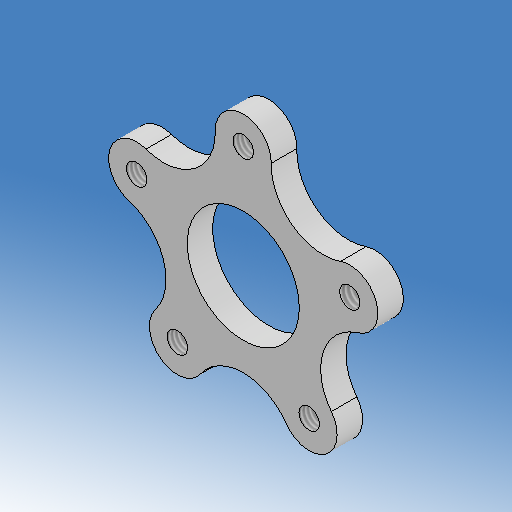
# Autodesk Inventor part: panel_flange
Saved by Autodesk Inventor 2025 (Build 290162000, 162)
## iProperties
Created: 2023-11-12
Part Number: panel_flange
Material: Generic
Document SubType Name: Modeling
Designer: ralph
Density: 1 g/cm^3
Appearance: Default
Author: ralph
Autodesk Inventor part; units mm, degrees
ref_plane "YZ Plane" through (0, 0, 0) normal (1, 0, 0) x (0, 1, 0)
ref_plane "XZ Plane" through (0, 0, 0) normal (0, 1, 0) x (-1, 0, 0)
ref_plane "XY Plane" through (0, 0, 0) normal (0, 0, 1) x (1, 0, 0)
sketch "Sketch1" plane through (0, 0, 0) normal (0, 0, 1) x (1, 0, 0)
  circle A0 centre (0, 0) radius 13.97
  circle A1 centre (0, 0) radius 34.925
  circle A2 centre (0, 0) radius 27.94
  point P0 (0, 27.94)
  point P1 (-26.5725, 8.6339)
  point P2 (-16.4227, -22.6039)
  point P3 (16.4227, -22.6039)
  point P4 (26.5725, 8.6339)
  dimension "d2" = 55.88
  dimension "d0" = 27.94
  dimension "d1" = 69.85
  dimension "d5" = 360
  constraints: 5 coincident, 2 centre point, 1 vertical alignment, 11 other
  measures "d0" diameter of A0
  measures "d1" diameter of A1
extrude "Extrusion1" add sketch "Sketch1" along normal blind 6.35 contours A1 | A2
hole "Hole1" at (0, 27.94, 0) at (-26.5725, 8.6339, 0) at (-16.4227, -22.6039, 0) at (16.4227, -22.6039, 0) at (26.5725, 8.6339, 0) direction (0, 0, 1) diameter 5.1054 end through all
thread "Thread1" size "1/4-20 UNC" class "2B" standard "ANSI Unified Screw Threads" full length
thread "Thread2" size "12-24 UNC" class "2B" standard "ANSI Unified Screw Threads" full length
thread "Thread3" size "12-24 UNC" class "2B" standard "ANSI Unified Screw Threads" full length
thread "Thread4" size "12-24 UNC" class "2B" standard "ANSI Unified Screw Threads" full length
thread "Thread5" size "12-24 UNC" class "2B" standard "ANSI Unified Screw Threads" full length
sketch "Sketch2" plane through (0, 0, 6.35) normal (0, 0, 1) x (1, 0, 0)
  circle A0 centre (0, 27.94) radius 2.5527 projected
  circle A1 centre (-26.5725, 8.6339) radius 2.5527 projected
  circle A2 centre (-16.4227, -22.6039) radius 2.5527 projected
  circle A3 centre (16.4227, -22.6039) radius 2.5527 projected
  circle A4 centre (26.5725, 8.6339) radius 2.5527 projected
  circle A5 centre (-26.5725, 8.6339) radius 6.985
  circle A6 centre (0, 27.94) radius 6.985
  circle A7 centre (26.5725, 8.6339) radius 6.985
  circle A8 centre (16.4227, -22.6039) radius 6.985
  circle A9 centre (-16.4227, -22.6039) radius 6.985
  circle A10 centre (0, 0) radius 34.925 projected
  circle A11 centre (0, 0) radius 20.955
  arc A12 (-24.2449, 15.2197) -> (-6.9827, 27.7615) centre (-19.9294, 27.4305) ccw
  arc A13 (-21.9669, -18.3552) -> (-28.5605, 1.9378) centre (-32.2464, -10.4775) ccw
  arc A14 (10.6686, -26.5638) -> (-10.6686, -26.5638) centre (0, -33.9059) ccw
  arc A15 (28.5605, 1.9378) -> (21.9669, -18.3552) centre (32.2464, -10.4775) ccw
  arc A16 (6.9827, 27.7615) -> (24.2449, 15.2197) centre (19.9294, 27.4305) ccw
  point P0 (-28.5605, 1.9378)
  point P1 (-33.2156, 10.7924)
  point P2 (-20.5284, -28.2549)
  point P3 (-21.9669, -18.3552)
  point P4 (0, 34.925)
  point P5 (33.2156, 10.7924)
  point P6 (6.9827, 27.7615)
  point P7 (21.9669, -18.3552)
  point P8 (20.5284, -28.2549)
  point P9 (28.5605, 1.9378)
  point P10 (-10.6686, -26.5638)
  point P11 (10.6686, -26.5638)
  dimension "d29" = 360
  constraints: 10 point on circle, 9 centre point, 2 equal radius, 1 coincident, 1 tangent, 32 other
extrude "Extrusion2" cut sketch "Sketch2" against normal blind 25.4 contours A5 A10 A6 A12 | A5 A13 A9 A10 | A10 A7 A16 A6 | A9 A14 A8 A10 | A10 A8 A15 A7
body "Solid1"
